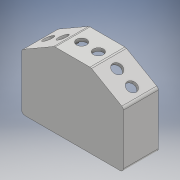
# Autodesk Inventor part: HousingBase
Saved by Autodesk Inventor 2017 (Build 210142000, 142)
## iProperties
Created: 2018-02-26
Part Number: HousingBase
Material: Generic
Document SubType Name: Modeling
Designer: tamer
Density: 1 g/cm^3
Appearance: Default
Author: tamer
## iProperties of the stored document HousingBase_3DPrint.ipt
Created: 2018-03-14
Part Number: HousingBase_3DPrint
Material: Generic
Document SubType Name: Modeling
Designer: Tamer
Density: 1 g/cm^3
Appearance: Default
Author: Tamer
Autodesk Inventor part; units mm, degrees
note: some values were not read from the file. Chosen so that the rebuilt part matches the saved one: side of "Thicken1".
ref_plane "YZ Plane" through (0, 0, 0) normal (1, 0, 0) x (0, 1, 0)
ref_plane "XZ Plane" through (0, 0, 0) normal (0, 1, 0) x (-1, 0, 0)
ref_plane "XY Plane" through (0, 0, 0) normal (0, 0, 1) x (1, 0, 0)
sketch "Sketch1" plane through (0, 0, 0) normal (0, 1, 0) x (-1, 0, 0)
  line L0 (0, 0) -> (0, 80)
  line L1 (0, 80) -> (-47.6314, 107.5)
  line L2 (-47.6314, 107.5) -> (-102.6314, 107.5)
  line L3 (-102.6314, 107.5) -> (-150.2628, 80)
  line L4 (-150.2628, 80) -> (-150.2628, 0)
  line L5 (-150.2628, 0) -> (0, 0)
  dimension "d0" = 80
  dimension "d1" = 55
  dimension "d2" = 120
  dimension "d3" = 55
  dimension "d4" = 55
  constraints: 12 end point, 2 perpendicular, 1 horizontal, 1 vertical
  measures "d0" distance of L0.start L0.end
  measures "d1" distance of L0.end L1.end
  measures "d2" angle of L1 L0
  measures "d3" distance of L1.end L2.end
  measures "d4" distance of L2.end L3.end
surface extrude "ExtrusionSrf1" sketch "Sketch1" against normal blind 50 shown no curves L0 L1 L2 L3 L4 L5
thicken "Thicken1" operation new thickness 5 both sides no extend neighbours no toward (-1, 0, 0) faces at (0, -16.6667, 26.6667) (15.8771, -16.6667, 89.1667) (65.9647, -16.6667, 107.5) (118.5085, -16.6667, 98.3333) (150.2628, -16.6667, 53.3333) (100.1752, -16.6667, 0)
sketch "Sketch2" plane through (-5, -50, -5) normal (0, -1, 0) x (1, 0, 0)
  line L0 (0, 87.8868) -> (0, 0) projected
  line L1 (0, 0) -> (0, 87.8868)
  line L2 (51.2917, 117.5) -> (108.9711, 117.5) projected
  line L3 (0, 87.8868) -> (51.2917, 117.5)
  line L4 (51.2917, 117.5) -> (108.9711, 117.5)
  line L5 (160.2628, 0) -> (160.2628, 87.8868) projected
  line L6 (108.9711, 117.5) -> (160.2628, 87.8868)
  line L7 (160.2628, 87.8868) -> (160.2628, 0)
  line L8 (160.2628, 0) -> (0, 0)
  point P0 (5, 5)
  constraints: 12 end point, 3 collinear, 1 perpendicular
extrude "Base" add sketch "Sketch2" along normal blind 5
sketch "Sketch3" plane through (-5, -50, -5) normal (0, 1, 0) x (1, 0, 0)
  line L0 (5, -5) -> (155.2628, -5) projected
  line L1 (90.5, -51) -> (90.5, -61.5)
  line L2 (5, -5) -> (5, -85) projected
  line L3 (90.5, -61.5) -> (80, -61.5)
  line L4 (5, -85) -> (5, -5) projected
  line L5 (90.5, -51) -> (92.5, -51)
  line L6 (92.5, -51) -> (92.5, -63.5)
  line L7 (92.5, -63.5) -> (80, -63.5)
  line L8 (80, -63.5) -> (80, -61.5)
  dimension "d12" = 2
  dimension "d13" = 10.5
  dimension "d14" = 12.5
  dimension "d15" = 12.5
  constraints: 12 end point, 3 perpendicular, 2 vertical, 1 horizontal
  measures "d12" distance of L1.start L5.end
  measures "d13" distance between parallel lines of L3 L5
  measures "d14" distance of L5.end L6.end
  measures "d15" distance of L6.end L7.end
extrude "Pi Holder" add sketch "Sketch3" along normal blind 4
sketch "Sketch4" plane through (-5, -55, 82.8868) normal (-0.5, 0, 0.8660254) x (0.8660254, 0, 0.5)
  line L0 (-43.9434, 55) -> (0, 55) projected
  line L1 (59.2265, 55) -> (59.2265, 0) projected
  line L2 (0, 55) -> (59.2265, 55)
  line L3 (0, 55) -> (0, 0)
  line L4 (-43.9434, 0) -> (94.8483, 0) projected
  line L5 (93.0181, 55) -> (-37.1132, 55) projected
  line L6 (0, 55) -> (0, 0) projected
  line L7 (0, 27.5) -> (59.2265, 27.5)
  circle A0 centre (42.8632, 27.5) radius 8
  circle A1 centre (16.3632, 27.5) radius 8
  line L8 (0, 55) -> (59.2265, 55) projected
  line L9 (29.6132, 55) -> (29.6132, 0)
  dimension "d18" = 16
  dimension "d19" = 16
  dimension "d20" = 26.5
  dimension "d36" = 26.5
  constraints: 8 end point, 4 point on line, 3 midpoint, 2 centre point, 2 vertical, 1 perpendicular
  measures "d18" diameter of A0
  measures "d19" diameter of A1
  measures "d20" distance of A0.centre A1.centre
  measures "d36" diameter of A0.centre L9
extrude "Sonar Holes 1" cut sketch "Sketch4" against normal blind 10 contours A0 L7 | L7 A0 | A1 L7 | L7 A1
sketch "Sketch5" plane through (46.2917, 0, 112.5) normal (0, 0, 1) x (1, 0, 0)
  line L0 (1.3397, 0) -> (56.3397, 0) projected
  line L1 (28.8397, 0) -> (28.8397, -55)
  line L2 (-51.2917, -55) -> (108.9711, -55) projected
  line L3 (0, 0) -> (0, -55) projected
  line L4 (0, -27.5) -> (57.6795, -27.5)
  line L5 (57.6795, 0) -> (57.6795, -55) projected
  circle A0 centre (42.0897, -27.5) radius 8
  circle A1 centre (15.5897, -27.5) radius 8
  point P0 (-46.2917, 0)
  dimension "d24" = 16
  dimension "d25" = 16
  dimension "d26" = 26.5
  dimension "d27" = 26.5
  constraints: 4 end point, 4 midpoint, 2 centre point, 2 point on line
  measures "d24" diameter of A0
  measures "d25" diameter of A1
  measures "d26" distance of A0.centre A1.centre
  measures "d27" diameter of A0.centre L1
extrude "Sonar Holes 2" cut sketch "Sketch5" against normal blind 10 contours A1 L4 | L4 A1 | A0 L4 | L4 A0
sketch "Sketch6" plane through (103.9711, -55, 112.5) normal (0.5, 0, 0.8660254) x (0.8660254, 0, -0.5)
  line L0 (96.3397, 55) -> (-33.7917, 55) projected
  line L1 (-35.6218, 0) -> (103.1699, 0) projected
  line L2 (0, 55) -> (0, 0) projected
  line L3 (0, 27.5) -> (59.2265, 27.5)
  line L4 (59.2265, 55) -> (59.2265, 0) projected
  circle A0 centre (42.8632, 27.5) radius 8
  circle A1 centre (16.3632, 27.5) radius 8
  line L5 (0, 55) -> (59.2265, 55) projected
  line L6 (29.6132, 55) -> (29.6132, 0)
  line L7 (59.2265, 0) -> (0, 0) projected
  dimension "d30" = 16
  dimension "d31" = 16
  dimension "d32" = 26.5
  dimension "d37" = 26.5
  constraints: 4 end point, 4 midpoint, 2 centre point, 2 point on line
  measures "d30" diameter of A0
  measures "d31" diameter of A1
  measures "d32" distance of A1.centre A0.centre
  measures "d37" diameter of A1.centre L6
extrude "Sonar Holes 3" cut sketch "Sketch6" against normal blind 10 contours A0 L3 | L3 A0 | A1 L3 | L3 A1
sketch "Sketch7" plane through (47.6314, -50, 107.5) normal (0.5, 0, -0.8660254) x (-0.8660254, 0, -0.5)
  line L0 (55, 50) -> (0, 50) projected
  line L1 (27.5, 50) -> (27.5, 0)
  line L2 (0, 0) -> (55, 0) projected
  line L3 (0, 50) -> (0, 0) projected
  line L4 (55, 50) -> (55, 0) projected
  line L5 (0, 22.5394) -> (55.0964, 22.5394)
  line L6 (5.7735, 22.5394) -> (5.7735, 27.5394)
  line L7 (50.7735, 22.5394) -> (50.7735, 27.5394)
  circle A0 centre (15.0235, 22.5) radius 8 projected
  circle A1 centre (41.5235, 22.5) radius 8 projected
  line L8 (5.7735, 22.5394) -> (5.7735, 17.5394)
  line L9 (50.7735, 22.5394) -> (50.7735, 17.5394)
  line L10 (5.7735, 27.5394) -> (3.7735, 27.5394)
  line L11 (3.7735, 27.5394) -> (3.7735, 17.5394)
  line L12 (3.7735, 17.5394) -> (5.7735, 17.5394)
  line L13 (50.7735, 27.5394) -> (52.7735, 27.5394)
  line L14 (52.7735, 27.5394) -> (52.7735, 17.5394)
  line L15 (52.7735, 17.5394) -> (50.7735, 17.5394)
  point P0 (95, 50)
  dimension "d38" = 45
  dimension "d39" = 9.25
  dimension "d40" = 9.25
  dimension "d46" = 2
  dimension "d47" = 2
  constraints: 24 end point, 5 perpendicular, 4 point on line, 3 vertical, 2 horizontal, 2 midpoint
  measures "d38" distance between parallel lines of L7 L6
  measures "d39" distance from line of L6 A0.centre
  measures "d40" distance from line of L7 A1.centre
  measures "d46" distance of L6.end L10.end
  measures "d47" distance of L7.end L13.end
extrude "Sonar Sidebars 1" add sketch "Sketch7" along normal blind 3 contours L14 L15 L9 L5 | L5 L7 L13 L14 | L11 L10 L6 L5 | L5 L8 L12 L11
chamfer "Chamfer1" distance 3 angle 45 2 edges at (44.9974, -32.4606, 102.5152) (4.2942, -32.4606, 79.0152)
sketch "Sketch8" plane through (102.6314, 0, 107.5) normal (0, 0, -1) x (-1, 0, 0)
  line L0 (55, 0) -> (0, 0) construction
  line L1 (27.5, 0) -> (27.5, -50) construction
  line L2 (0, -50) -> (55, -50) construction
  line L3 (0, 0) -> (0, -50) construction
  line L4 (55, 0) -> (55, -50) construction
  line L5 (0, -27.5) -> (55, -27.5) construction
  line L6 (5, -27.5) -> (5, -22.5)
  line L7 (50, -27.5) -> (50, -22.5)
  circle A0 centre (14.25, -27.5) radius 8 projected
  circle A1 centre (40.75, -27.5) radius 8 projected
  line L8 (5, -27.5) -> (5, -32.5)
  line L9 (5, -32.5) -> (3, -32.5)
  line L10 (3, -32.5) -> (3, -22.5)
  line L11 (3, -22.5) -> (5, -22.5)
  line L12 (50, -22.5) -> (52, -22.5)
  line L13 (52, -22.5) -> (52, -32.5)
  line L14 (52, -32.5) -> (50, -32.5)
  line L15 (50, -32.5) -> (50, -27.5)
  point P0 (102.6314, 0)
  dimension "d53" = 5
  dimension "d54" = 5
  dimension "d55" = 45
  dimension "d56" = 9.25
  dimension "d57" = 9.25
  dimension "d58" = 5
  dimension "d59" = 2
  dimension "d60" = 2
  dimension "d61" = 10
  constraints: 24 end point, 7 point on line, 5 perpendicular, 3 vertical, 2 midpoint
  measures "d53" distance of L6.start L6.end
  measures "d54" distance of L7.start L7.end
  measures "d55" distance between parallel lines of L7 L6
  measures "d56" distance from line of A0.centre L6
  measures "d57" distance from line of A1.centre L7
  measures "d58" distance of L6.start L8.end
  measures "d59" distance of L8.end L9.end
  measures "d60" distance of L7.end L12.end
  measures "d61" distance of L12.end L13.end
extrude "Sonar Sidebars 2" add sketch "Sketch8" along normal blind 3 contours L8 L9 L10 L11 L6 | L7 L12 L13 L14 L15
chamfer "Chamfer2" distance 3 angle 45 2 edges at (98.6314, -32.5, 104.5) (51.6314, -32.5, 104.5)
sketch "Sketch9" plane through (150.2628, -50, 80) normal (-0.5, 0, -0.8660254) x (-0.8660254, 0, 0.5)
  line L0 (4.6443, 22.5) -> (55, 22.5) construction
  line L1 (55, 50) -> (55, 0) construction
  line L2 (0, 50) -> (0, 0) construction
  line L3 (4.6443, 22.5) -> (0, 22.5) construction
  line L4 (4.2265, 22.5) -> (4.2265, 27.5)
  line L5 (49.2265, 22.5) -> (49.2265, 27.5)
  circle A0 centre (39.9765, 22.5) radius 8 projected
  circle A1 centre (13.4765, 22.5) radius 8 projected
  line L6 (55, 50) -> (0, 50) projected
  line L7 (0, 50) -> (0, 0) projected
  line L8 (0, 0) -> (55, 0) projected
  line L9 (55, 50) -> (55, 0) projected
  line L10 (4.2265, 22.5) -> (4.2265, 17.5)
  line L11 (4.2265, 17.5) -> (2.2265, 17.5)
  line L12 (2.2265, 17.5) -> (2.3223, 27.5182)
  line L13 (2.3223, 27.5182) -> (4.2265, 27.5)
  line L14 (49.2265, 22.5) -> (49.2265, 17.5)
  line L15 (49.2265, 17.5) -> (51.2265, 17.5)
  line L16 (51.2265, 17.5) -> (51.2265, 27.5)
  line L17 (51.2265, 27.5) -> (49.2265, 27.5)
  point P0 (90.1314, 50)
  dimension "d67" = 5
  dimension "d68" = 5
  dimension "d69" = 45
  dimension "d70" = 9.25
  dimension "d71" = 5
  dimension "d72" = 2
  dimension "d74" = 5
  dimension "d75" = 2
  constraints: 24 end point, 7 perpendicular, 4 point on line, 3 vertical, 1 horizontal
  measures "d67" distance of L4.start L4.end
  measures "d68" distance of L5.start L5.end
  measures "d69" distance between parallel lines of L5 L4
  measures "d70" distance from line of A1.centre L4
  measures "d71" distance of L4.start L10.end
  measures "d72" distance of L10.end L11.end
  measures "d74" distance of L5.start L14.end
  measures "d75" distance of L14.end L15.end
extrude "Sonar Sidebars 3" add sketch "Sketch9" along normal blind 3 contours L10 L11 L12 L13 L4 | L5 L17 L16 L15 L14
chamfer "Chamfer3" distance 3 angle 45 2 edges at (145.9686, -32.5, 79.0152) (105.2654, -32.5, 102.5152)
fillet "Fillet1" radius 5 6 edges at (46.2917, -27.5, 112.5) (103.9711, -27.5, 112.5) (-5, -27.5, 82.8868) (155.2628, -27.5, 82.8868) (155.2628, -27.5, -5) (-5, -27.5, -5)
sketch "Sketch11" plane through (0, 0, -5) normal (0, 1, 0) x (1, 0, 0)
  line L0 (102.6314, -112.5) -> (47.6314, -112.5) construction
  line L1 (75.1314, -112.5) -> (75.1314, -117.5) construction
  line L2 (47.6314, -117.5) -> (102.6314, -117.5) construction
  circle A0 centre (75.1314, -115) radius 1.15
  line L3 (-5, -5) -> (-5, -85) construction
  line L4 (-5, -85) -> (0, -85) construction
  line L5 (0, -5) -> (-5, -5) construction
  line L6 (-2.5, -5) -> (-2.5, -85) construction
  circle A1 centre (-2.5, -85) radius 1.15
  circle A2 centre (-2.5, -5) radius 1.15
  arc A3 (152.7628, -89.3301) -> (155.2628, -85) centre (150.2628, -85) ccw construction
  line L7 (150.2628, -85) -> (155.2628, -85) construction
  line L8 (155.2628, -85) -> (155.2628, -5) construction
  line L9 (150.2628, -5) -> (155.2628, -5) construction
  line L10 (152.7628, -5) -> (152.7628, -85) construction
  circle A4 centre (152.7628, -5) radius 1.15
  circle A5 centre (152.7628, -85) radius 1.15
  dimension "d82" = 2.3
  dimension "d83" = 2.3
  dimension "d84" = 2.3
  dimension "d85" = 2.3
  dimension "d86" = 2.3
  constraints: 14 end point, 7 midpoint, 5 centre point, 4 coincident, 4 horizontal
  measures "d82" diameter of A0
  measures "d83" diameter of A1
  measures "d84" diameter of A2
  measures "d85" diameter of A4
  measures "d86" diameter of A5
extrude "Screw Holes" cut sketch "Sketch11" against normal blind 5
sketch "Sketch12" plane through (150.2628, 0, -5) normal (0, 0, -1) x (-1, 0, 0)
  line L0 (0, 0) -> (150.2628, 0) construction
  line L1 (75.1314, 0) -> (75.1314, -55) construction
  line L2 (150.2628, -55) -> (0, -55) construction
  line L3 (75.1314, 0) -> (65.1314, 0)
  line L4 (65.1314, 0) -> (65.1314, -5)
  line L5 (65.1314, -5) -> (85.1314, -5)
  line L6 (73.9814, -5) -> (76.2814, -5) projected
  line L7 (85.1314, -5) -> (85.1314, 0)
  line L8 (85.1314, 0) -> (75.1314, 0)
  dimension "d99" = 10
  dimension "d100" = 5
  dimension "d101" = 20
  constraints: 12 end point, 2 collinear, 2 midpoint, 2 perpendicular, 2 point on line
  measures "d99" distance of L1.start L3.end
  measures "d100" distance of L3.end L4.end
  measures "d101" distance of L4.end L5.end
extrude "Wiring Slit" cut sketch "Sketch12" against normal blind 5
sketch "Sketch13" plane through (-5, -50, -5) normal (0, 1, 0) x (1, 0, 0)
  line L0 (5, -5) -> (155.2628, -5) construction
  line L1 (217.8251, -5) -> (-40.768, -5) construction
  line L2 (5, 13.1586) -> (5, -114.6539) construction
  line L3 (90.5, -126.5262) -> (90.5, 16.4977) construction
  line L4 (195.75, -61.5) -> (-35.7594, -61.5) construction
  line L5 (5, -85) -> (5, -5) construction
  line L6 (5, -5) -> (5, -8.5) construction
  line L7 (5, -8.5) -> (8.5, -8.5) construction
  circle A0 centre (8.5, -8.5) radius 1.15
  line L8 (5, -61.5) -> (8.5, -61.5) construction
  line L9 (8.5, -61.5) -> (8.5, -58) construction
  circle A1 centre (8.5, -58) radius 1.15
  line L10 (90.5, -51) -> (90.5, -61.5) construction
  line L11 (90.5, -61.5) -> (90.5, -58) construction
  circle A2 centre (66.5, -58) radius 1.15
  line L12 (155.2628, -5) -> (90.1314, -5) construction
  line L13 (90.5, -5) -> (90.5, -8.5) construction
  line L14 (90.5, -8.5) -> (66.5, -8.5) construction
  circle A3 centre (66.5, -8.5) radius 1.15
  dimension "d104" = 3.5
  dimension "d105" = 3.5
  dimension "d106" = 2.3
  dimension "d107" = 3.5
  dimension "d108" = 2.3
  dimension "d110" = 2.3
  dimension "d113" = 58
  dimension "d114" = 58
  constraints: 22 end point, 8 point on line, 4 centre point, 3 coincident, 3 horizontal, 2 vertical, 1 perpendicular
  measures "d104" distance of L0.start L6.end
  measures "d105" distance of L6.end L7.end
  measures "d106" diameter of A0
  measures "d107" distance of L8.end L9.end
  measures "d108" diameter of A1
  measures "d110" diameter of A2
  measures "d113" distance of A2.centre A1.centre
  measures "d114" distance of L14.end L7.end
extrude "Pi Holes" cut sketch "Sketch13" against normal blind 3
body "Solid1"
body "Srf1"
